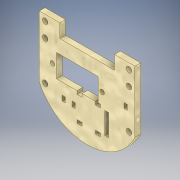
# Autodesk Inventor part: PixyCamGimbal Body
Saved by Autodesk Inventor 2017 (Build 210142000, 142)
## iProperties
Created: 2016-12-06
Part Number: PixyCamGimbal Body
Material: Generic
Document SubType Name: Modeling
Designer: PLTW
Density: 1 g/cm^3
Appearance: Fine - Cream
Author: PLTW
Autodesk Inventor part; units mm, degrees
ref_plane "YZ Plane" through (0, 0, 0) normal (1, 0, 0) x (0, 1, 0)
ref_plane "XZ Plane" through (0, 0, 0) normal (0, 1, 0) x (-1, 0, 0)
ref_plane "XY Plane" through (0, 0, 0) normal (0, 0, 1) x (1, 0, 0)
sketch "Sketch1" plane through (0, 0, 0) normal (0, 0, 1) x (1, 0, 0)
  arc A0 (-26.67, -12.5235) -> (26.67, -12.5235) centre (0, 0) ccw
  line L0 (-26.67, -12.5235) -> (-26.67, 21.7665)
  line L1 (-26.67, 21.7665) -> (-15.24, 21.7665)
  line L2 (-15.24, 21.7665) -> (-15.24, 14.1465)
  line L3 (-15.24, 14.1465) -> (15.24, 14.1465)
  line L4 (15.24, 14.1465) -> (15.24, 21.7665)
  line L5 (15.24, 21.7665) -> (26.67, 21.7665)
  line L6 (26.67, 21.7665) -> (26.67, -12.5235)
  line L7 (-17.018, 6.5265) -> (6.096, 6.5265)
  line L8 (6.096, 6.5265) -> (6.096, -6.1735)
  line L9 (6.096, -6.1735) -> (-17.018, -6.1735)
  line L10 (-17.018, -6.1735) -> (-17.018, 6.5265)
  line L11 (-5.588, -6.1735) -> (-2.794, -6.1735)
  line L12 (-2.794, -6.1735) -> (-2.794, -7.9515)
  line L13 (-2.794, -7.9515) -> (-5.588, -7.9515)
  line L14 (-5.588, -7.9515) -> (-5.588, -6.1735)
  line L15 (4.572, -6.1735) -> (7.366, -6.1735)
  line L16 (7.366, -6.1735) -> (7.366, -7.9515)
  line L17 (7.366, -7.9515) -> (4.572, -7.9515)
  line L18 (4.572, -7.9515) -> (4.572, -6.1735)
  line L19 (9.906, -7.9515) -> (11.938, -7.9515)
  line L20 (11.938, -7.9515) -> (11.938, -20.1435)
  line L21 (11.938, -20.1435) -> (9.906, -20.1435)
  line L22 (9.906, -20.1435) -> (9.906, -7.9515)
  line L23 (-5.588, -20.1435) -> (-2.794, -20.1435)
  line L24 (-2.794, -20.1435) -> (-2.794, -21.9215)
  line L25 (-2.794, -21.9215) -> (-5.588, -21.9215)
  line L26 (-5.588, -21.9215) -> (-5.588, -20.1435)
  line L27 (-8.382, -12.5235) -> (-6.604, -12.5235)
  line L28 (-6.604, -12.5235) -> (-6.604, -15.3175)
  line L29 (-6.604, -15.3175) -> (-8.382, -15.3175)
  line L30 (-8.382, -15.3175) -> (-8.382, -12.5235)
  line L31 (-13.97, -12.5235) -> (-12.192, -12.5235)
  line L32 (-12.192, -12.5235) -> (-12.192, -15.3175)
  line L33 (-12.192, -15.3175) -> (-13.97, -15.3175)
  line L34 (-13.97, -15.3175) -> (-13.97, -12.5235)
  line L35 (20.574, 1.1925) -> (22.352, 1.1925)
  line L36 (22.352, 1.1925) -> (22.352, -1.6015)
  line L37 (22.352, -1.6015) -> (20.574, -1.6015)
  line L38 (20.574, -1.6015) -> (20.574, 1.1925)
  line L39 (4.572, -20.1435) -> (7.366, -20.1435)
  line L40 (7.366, -20.1435) -> (7.366, -21.9215)
  line L41 (7.366, -21.9215) -> (4.572, -21.9215)
  line L42 (4.572, -21.9215) -> (4.572, -20.1435)
  circle A1 centre (-23.368, 18.4645) radius 1.524
  circle A2 centre (-23.368, 10.3365) radius 1.524
  circle A3 centre (-23.368, -11.5075) radius 1.524
  circle A4 centre (-19.304, 0.1765) radius 1.27
  circle A5 centre (8.382, 0.1765) radius 1.27
  circle A6 centre (23.368, 18.4645) radius 1.524
  circle A7 centre (23.368, 10.3365) radius 1.524
  circle A8 centre (23.368, -11.5075) radius 1.524
  dimension "d0" = 29.464
  dimension "d1" = 34.29
  dimension "d2" = 11.43
  dimension "d3" = 7.62
  dimension "d4" = 30.48
  dimension "d5" = 2.794
  dimension "d6" = 12.7
  dimension "d7" = 23.114
  dimension "d8" = 7.62
  dimension "d9" = 9.652
  dimension "d10" = 1.778
  dimension "d11" = 12.954
  dimension "d12" = 4.318
  dimension "d13" = 12.192
  dimension "d14" = 7.366
  dimension "d15" = 2.032
  dimension "d16" = 2.54
  dimension "d17" = 1.27
  dimension "d18" = 1.016
  dimension "d19" = 4.572
  dimension "d20" = 3.81
  dimension "d21" = 3.048
  dimension "d22" = 2.54
  dimension "d23" = 3.302
  dimension "d24" = 3.302
  dimension "d25" = 3.302
  dimension "d26" = 3.302
  dimension "d27" = 8.128
  dimension "d28" = 21.844
  dimension "d29" = 2.286
  dimension "d30" = 2.286
  dimension "d31" = 6.35
  constraints: 86 end point, 18 parallel, 14 perpendicular, 12 equal length, 9 centre point, 9 horizontal, 7 horizontal alignment, 7 point on line, 6 equal radius, 6 vertical alignment, 2 point on circle, 1 coincident, 1 vertical
  measures "d0" radius of A0
  measures "d1" distance of L0.start L0.end
  measures "d2" distance of L0.end L1.end
  measures "d3" distance of L1.end L2.end
  measures "d4" distance of L2.end L3.end
  measures "d5" distance of L12.end L13.end
  measures "d6" distance of L9.end L7.start
  measures "d7" distance of L7.start L7.end
  measures "d8" distance between parallel lines of L7 L3
  measures "d9" distance between parallel lines of L0 L10
  measures "d10" distance of L35.start L35.end
  measures "d11" distance between parallel lines of L35 L3
  measures "d12" distance between parallel lines of L6 L36
  measures "d13" distance between parallel lines of L23 L13
  measures "d14" distance of L15.start L11.end
  measures "d15" distance of L19.start L19.end
  measures "d16" distance between parallel lines of L22 L16
  measures "d17" distance between parallel lines of L8 L16
  measures "d18" distance from line of L13.end L28
  measures "d19" distance between parallel lines of L27 L13
  measures "d20" distance between parallel lines of L30 L32
  measures "d21" diameter of A1
  measures "d22" diameter of A4
  measures "d23" distance from line of L1 A1.centre
  measures "d24" distance from line of L0 A1.centre
  measures "d25" distance from line of L6 A6.centre
  measures "d26" distance from line of L5 A6.centre
  measures "d27" distance of A1.centre A2.centre
  measures "d28" distance of A3.centre A2.centre
  measures "d29" distance from line of L8 A5.centre
  measures "d30" distance from line of L10 A4.centre
  measures "d31" distance from line of L9 A5.centre
extrude "Extrusion1" add sketch "Sketch1" along normal blind 3.175
body "Solid1"
